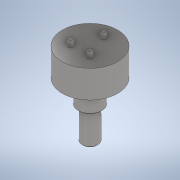
# Autodesk Inventor part: TT_Electronics_Encoder_6127V1A360L.5FS
Saved by Autodesk Inventor 2020 (Build 240168000, 168)
## iProperties
Created: 2019-06-03
Part Number: TT_Electronics_Encoder_6127V1A360L.5FS
Material: Steel, Alloy
Document SubType Name: Modeling
Designer: Connor
Density: 7.73 g/cm^3
Appearance: Semi-Polished
Author: Connor
Autodesk Inventor part; units mm, degrees
ref_plane "YZ Plane" through (0, 0, 0) normal (1, 0, 0) x (0, 1, 0)
ref_plane "XZ Plane" through (0, 0, 0) normal (0, 1, 0) x (-1, 0, 0)
ref_plane "XY Plane" through (0, 0, 0) normal (0, 0, 1) x (1, 0, 0)
sketch "Sketch1" plane through (0, 0, 0) normal (0, 0, 1) x (1, 0, 0)
  line L0 (0, 0) -> (3.1712, 0)
  line L1 (3.1712, 0) -> (3.1712, 11.8618)
  line L2 (3.1712, 11.8618) -> (0, 11.8618)
  line L3 (0, 11.8618) -> (0, 0)
  line L4 (0, 11.8618) -> (2.9028, 11.8618)
  line L5 (2.9028, 11.8618) -> (2.9028, 12.7)
  line L6 (2.9028, 12.7) -> (0, 12.7)
  line L7 (0, 12.7) -> (0, 11.8618)
  line L8 (0, 12.7) -> (4.7625, 12.7)
  line L9 (4.7625, 12.7) -> (4.7625, 20.7264)
  line L10 (4.7625, 20.7264) -> (0, 20.7264)
  line L11 (0, 20.7264) -> (0, 12.7)
  line L12 (0, 20.7264) -> (5.1562, 20.7264)
  line L13 (5.1562, 20.7264) -> (5.1562, 22.225)
  line L14 (5.1562, 22.225) -> (0, 22.225)
  line L15 (0, 22.225) -> (0, 20.7264)
  line L16 (0, 22.225) -> (11.1125, 22.225)
  line L17 (11.1125, 22.225) -> (11.1125, 33.274)
  line L18 (11.1125, 33.274) -> (0, 33.274)
  line L19 (0, 33.274) -> (0, 22.225)
  dimension "d0" = 22.225
  dimension "d1" = 9.525
  dimension "d2" = 1.4986
  dimension "d3" = 0.8382
  dimension "d4" = 3.1712
  dimension "d5" = 5.1562
  dimension "d6" = 11.049
  dimension "d7" = 11.1125
  dimension "d8" = 4.7625
  constraints: 40 end point, 10 parallel, 5 horizontal, 5 perpendicular
  measures "d0" distance between parallel lines of L0 L16
  measures "d1" distance between parallel lines of L8 L16
  measures "d2" distance of L12.end L13.end
  measures "d3" distance of L4.end L5.end
  measures "d4" distance of L0.start L0.end
  measures "d5" distance between parallel lines of L15 L13
  measures "d6" distance of L16.end L17.end
  measures "d7" distance of L17.end L18.end
  measures "d8" distance between parallel lines of L9 L11
revolve "Revolution1" add sketch "Sketch1" angle 360 about axis through (0, 33.274, 0) along (0, -1, 0)
chamfer "Chamfer1" distance 0.3969 angle 45 2 edges at (-3.1712, 0, 0) (-4.7625, 12.7, 0)
sketch "Sketch2" plane through (0, 22.225, 0) normal (0, -1, 0) x (1, 0, 0)
  circle A0 centre (0, -7.366) radius 0.7874
  circle A1 centre (0, 0) radius 11.1125 projected
  point P0 (0, 0)
  dimension "d13" = 1.5748
  dimension "d14" = 7.366
  constraints: 1 centre point, 1 vertical alignment
  measures "d13" diameter of A0
  measures "d14" distance of A1.centre A0.centre
extrude "Extrusion1" add sketch "Sketch2" along normal blind 1.5748 contours A0
sketch "Sketch3" plane through (0, 0, 0) normal (0, -1, 0) x (1, 0, 0)
  line L0 (-2.1671, -2.3152) -> (2.1671, -2.3152)
  circle A0 centre (0, 0) radius 3.1712 projected
  point P0 (0, 0)
  dimension "d18" = 5.4864
  constraints: 2 end point, 2 point on circle, 1 horizontal
extrude "Extrusion2" cut sketch "Sketch3" against normal blind 9.525 contours L0 A0 picked at (-0.5411, -2.4515)
sketch "Sketch4" plane through (0, 33.274, 0) normal (0, 1, 0) x (1, 0, 0)
  circle A0 centre (0, 0) radius 5.5245 construction
  circle A1 centre (3.9116, -3.9012) radius 0.889
  circle A2 centre (-3.9116, -3.9012) radius 0.889
  circle A3 centre (0, 5.5245) radius 0.889
  line L0 (3.9116, -3.9012) -> (-3.9116, -3.9012) construction
  line L1 (0, 0) -> (0, 11.1125) construction
  circle A4 centre (0, 0) radius 11.1125 construction
  dimension "d21" = 11.049
  dimension "d22" = 7.8232
  dimension "d23" = 1.778
  constraints: 4 centre point, 4 end point, 3 point on circle, 2 equal radius, 1 coincident, 1 horizontal, 1 point on line, 1 vertical, 1 vertical alignment, 1 other
  measures "d21" diameter of A0
  measures "d22" distance of L0.end L0.start
  measures "d23" diameter of A1
extrude "Extrusion3" add sketch "Sketch4" along normal blind 2.4892
body "Solid1"
